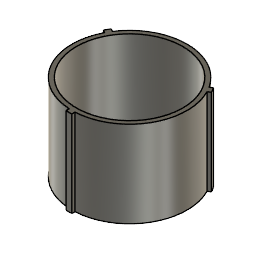
Final_flashpaper_chamber_inner (Autodesk Fusion 360 design; units mm, degrees)
part number: 2026-05-27-16-13-41-034
Autodesk Fusion 360 part; units mm, degrees
sketch "Sketch1" plane through (0, 0, 0) normal (0, 0, 1) x (1, 0, 0)
  circle A0 centre (0, 0) radius 20
  line L0 (1, -19.975) -> (1, -21.1)
  line L1 (1, -21.1) -> (-1, -21.1)
  line L2 (-1, -21.1) -> (-1, -19.975)
  line L3 (18.7731, 9.684) -> (17.7988, 9.1215)
  line L4 (17.7731, 11.416) -> (18.7731, 9.684)
  line L5 (16.7988, 10.8535) -> (17.7731, 11.416)
  line L6 (-17.7731, 11.416) -> (-16.7988, 10.8535)
  line L7 (-18.7731, 9.684) -> (-17.7731, 11.416)
  line L8 (-17.7988, 9.1215) -> (-18.7731, 9.684)
  dimension "d5" = 40
  dimension "d9" = 2
  dimension "d12" = 360
  constraint coincident A0.centre origin
  constraint parallel L0 L2
  constraint coincident A0 L0.start
  constraint coincident A0 L2.end
  measures "d5" diameter of A0
  measures "d9" distance of L0.end L1.end
extrude "Extrude2" add sketch "Sketch1" along normal blind 30 contours A0
shell "Shell2" thickness 1.5 removed faces 1 at (-4.9181, 4.3771, 30)
extrude "Extrude3" add sketch "Sketch1" along normal up to surface (30 mm away) contours A0 L3 L4 L5 | A0 L0 L1 L2 | A0 L6 L7 L8
